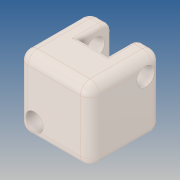
# Autodesk Inventor part: 方块2_beta
Saved by Autodesk Inventor 2019.1 (Build 231200000, 200)
## iProperties
Created: 2020-09-27
Part Number: 方块2_beta
Material: Generic
Document SubType Name: Modeling
Designer: 谢庆红冰
Density: 1 g/cm^3
Appearance: 缎光 - 亚麻
Author: 谢庆红冰
Autodesk Inventor part; units mm, degrees
ref_plane "YZ Plane" through (0, 0, 0) normal (1, 0, 0) x (0, 1, 0)
sketch "草图1" plane through (0, 0, 0) normal (0, 1, 0) x (-1, 0, 0)
  line L0 (-10, 10) -> (10, 10)
  line L1 (10, 10) -> (10, -10)
  line L2 (10, -10) -> (-10, -10)
  line L3 (-10, -10) -> (-10, 10)
  line L4 (-10, 10) -> (10, -10) construction
  line L5 (10, 10) -> (-10, -10) construction
  point P0 (0, 0)
  dimension "d0" = 20
  dimension "d1" = 20
  constraints: 12 end point, 2 midpoint, 2 parallel, 1 horizontal, 1 perpendicular
  measures "d0" distance of L0.end L1.end
  measures "d1" distance of L1.end L2.end
extrude "拉伸1" add sketch "草图1" along normal blind 20
ref_plane "工作平面1" through (0, 0, 10) normal (1, 0, 0) x (0, 0, -1)
sketch "草图6" plane through (0, 0, 0) normal (0, 0, 1) x (1, 0, 0)
  line L0 (10, 0) -> (-10, 0) construction
  line L1 (10, 0) -> (10, 20) construction
  line L2 (-10, 20) -> (10, 20) construction
  line L3 (-10, 0) -> (-10, 20) construction
  line L4 (-10, 20) -> (10, 0) construction
  line L5 (7.5, 12.5) -> (-2.5, 12.5)
  line L6 (-2.5, 12.5) -> (-2.5, 2.5)
  line L7 (-2.5, 2.5) -> (7.5, 2.5)
  line L8 (7.5, 2.5) -> (7.5, 12.5)
  line L9 (7.5, 12.5) -> (-2.5, 2.5) construction
  line L10 (-2.5, 12.5) -> (7.5, 2.5) construction
  point P0 (0, 0)
  point P1 (2.5, 7.5)
  dimension "d58" = 10
  dimension "d59" = 10
  constraints: 14 end point, 2 midpoint, 2 parallel, 1 horizontal, 1 perpendicular, 1 point on line
  measures "d58" distance of L7.end L6.end
  measures "d59" distance of L5.end L6.end
extrude "拉伸6" [suppressed]
sketch "草图2" plane through (0, 0, 10) normal (1, 0, 0) x (0, 0, -1)
  line L0 (20, 0) -> (0, 0) construction
  line L1 (20, 0) -> (20, 20) construction
  line L2 (0, 20) -> (20, 20) construction
  line L3 (0, 0) -> (0, 20) construction
  line L4 (20, 20) -> (20, 11)
  line L5 (20, 20) -> (11, 20)
  line L6 (20, 11) -> (11, 11)
  line L7 (11, 11) -> (11, 20)
  point P0 (10, 0)
  dimension "d4" = 9
  dimension "d5" = 9
  constraints: 9 end point, 2 perpendicular, 2 point on line
  measures "d4" distance of L4.end L1.end
  measures "d5" distance of L1.end L5.end
extrude "拉伸2" cut sketch "草图2" along normal mid plane 8
ref_plane "工作平面2" through (-10, 0, 0) normal (0, 0, 1) x (1, 0, 0)
sketch "草图3" plane through (-10, 0, 0) normal (0, 0, 1) x (1, 0, 0)
  line L0 (20, 0) -> (0, 0) construction
  line L1 (20, 0) -> (20, 20) construction
  line L2 (0, 20) -> (20, 20) construction
  line L3 (0, 0) -> (0, 20) construction
  line L4 (0, 0) -> (6, 0)
  line L5 (0, 0) -> (9, 0)
  line L6 (9, 0) -> (9, 9)
  line L7 (9, 9) -> (0, 9)
  line L8 (0, 9) -> (0, 0)
  point P0 (10, 0)
  dimension "d8" = 6
  dimension "d9" = 9
  dimension "d10" = 9
  constraints: 10 end point, 2 parallel, 1 horizontal, 1 perpendicular, 1 point on line
  measures "d8" distance of L0.end L4.end
  measures "d9" distance of L7.end L6.end
  measures "d10" distance of L5.end L6.end
extrude "拉伸3" cut sketch "草图3" along normal mid plane 8
sketch "草图4" plane through (-10, 0, 0) normal (0, 0, 1) x (1, 0, 0)
  line L0 (20, 0) -> (0, 0) construction
  line L1 (20, 0) -> (20, 20) construction
  line L2 (0, 20) -> (20, 20) construction
  line L3 (0, 0) -> (0, 20) construction
  line L4 (4.5, 6.5) -> (4.5, 2.5) construction
  line L5 (3.75, 5.75) -> (3.75, 3.25)
  arc A0 (3.75, 3.25) -> (5.25, 3.25) centre (4.5, 3.25) ccw
  arc A1 (5.25, 5.75) -> (3.75, 5.75) centre (4.5, 5.75) ccw
  line L6 (3.75, 5.75) -> (3.75, 3.25)
  line L7 (0, 0) -> (9, 0) construction
  line L8 (0, 9) -> (0, 0) construction
  line L9 (9, 9) -> (0, 9) construction
  line L10 (9, 0) -> (9, 9) construction
  line L11 (0, 9) -> (9, 0) construction
  line L12 (0, 0) -> (9.9155, 8.0845) construction
  line L13 (5.25, 3.25) -> (5.25, 5.75)
  line L14 (3.75, 5.75) -> (5.25, 5.75) construction
  line L15 (2.5, 4.5) -> (6.5, 4.5) construction
  line L16 (3.25, 3.75) -> (5.75, 3.75)
  line L17 (3.25, 3.75) -> (5.75, 3.75)
  arc A2 (5.75, 3.75) -> (5.75, 5.25) centre (5.75, 4.5) ccw
  arc A3 (3.25, 5.25) -> (3.25, 3.75) centre (3.25, 4.5) ccw
  line L18 (5.75, 5.25) -> (3.25, 5.25)
  line L19 (3.25, 3.75) -> (3.25, 5.25) construction
  circle A4 centre (4.5, 4.5) radius 2.5
  point P0 (10, 0)
  point P1 (3, 3)
  point P2 (3, 3)
  point P3 (3, 3)
  point P4 (4.5, 4.5)
  point P5 (3, 3)
  point P6 (3, 3)
  point P7 (3, 3)
  point P8 (3, 3)
  dimension "d42" = 0.75
  dimension "d43" = 0.75
  dimension "d44" = 2.5
  dimension "d45" = 1.5
  dimension "d46" = 0.75
  dimension "d47" = 0.75
  dimension "d48" = 2.5
  dimension "d49" = 1.5
  dimension "d66" = 5
  constraints: 24 end point, 12 point on circle, 5 centre point, 5 parallel, 4 point on line, 3 midpoint, 1 coincident, 1 horizontal
  measures "d42" radius of A1
  measures "d43" radius of A0
  measures "d44" distance of L13.start L13.end
  measures "d45" distance of L5.start L13.end
  measures "d46" radius of A3
  measures "d47" radius of A2
  measures "d48" distance of L18.start L19.end
  measures "d49" distance of L16.start L19.end
  measures "d66" diameter of A4
extrude "拉伸4" cut sketch "草图4" along normal through all both and the other way through all contours A1 L13 L18 L5 | L18 L13 L16 L5 | L5 L16 A3 L18 | L16 L13 A0 L5 | L18 A2 L16 L13 | A4
sketch "草图5" plane through (0, 0, 10) normal (1, 0, 0) x (0, 0, -1)
  line L0 (20, 0) -> (0, 0) construction
  line L1 (20, 0) -> (20, 20) construction
  line L2 (0, 20) -> (20, 20) construction
  line L3 (0, 0) -> (0, 20) construction
  line L4 (20, 20) -> (20, 11) construction
  line L5 (11, 20) -> (20, 20) construction
  line L6 (11, 11) -> (11, 20) construction
  line L7 (20, 11) -> (11, 11) construction
  line L8 (11, 20) -> (20, 11) construction
  line L9 (15.5, 17.5) -> (15.5, 13.5) construction
  line L10 (14.75, 16.75) -> (14.75, 14.25)
  line L11 (14.75, 16.75) -> (14.75, 14.25)
  arc A0 (14.75, 14.25) -> (16.25, 14.25) centre (15.5, 14.25) ccw
  arc A1 (16.25, 16.75) -> (14.75, 16.75) centre (15.5, 16.75) ccw
  line L12 (16.25, 14.25) -> (16.25, 16.75)
  line L13 (14.75, 16.75) -> (16.25, 16.75) construction
  line L14 (14.25, 14.75) -> (16.75, 14.75)
  line L15 (14.25, 14.75) -> (16.75, 14.75)
  line L16 (13.5, 15.5) -> (17.5, 15.5) construction
  line L17 (14.25, 14.75) -> (14.25, 16.25) construction
  line L18 (16.75, 16.25) -> (14.25, 16.25)
  arc A2 (16.75, 14.75) -> (16.75, 16.25) centre (16.75, 15.5) ccw
  arc A3 (14.25, 16.25) -> (14.25, 14.75) centre (14.25, 15.5) ccw
  line L19 (12.5, 12.5) -> (20, 20) construction
  circle A4 centre (15.5, 15.5) radius 2.5
  point P0 (10, 0)
  point P1 (7.5, 0)
  point P2 (3, 3)
  point P3 (3, 3)
  point P4 (3, 3)
  point P5 (3, 3)
  point P6 (3, 3)
  point P7 (3, 3)
  point P8 (3, 3)
  point P9 (3, 3)
  point P10 (16.25, 16.25)
  dimension "d50" = 0.75
  dimension "d51" = 0.75
  dimension "d52" = 2.5
  dimension "d53" = 1.5
  dimension "d54" = 0.75
  dimension "d55" = 0.75
  dimension "d56" = 2.5
  dimension "d57" = 1.5
  dimension "d65" = 5
  constraints: 24 end point, 12 point on circle, 5 centre point, 5 parallel, 4 midpoint, 4 point on line, 1 coincident, 1 horizontal
  measures "d50" radius of A1
  measures "d51" radius of A0
  measures "d52" distance of L12.start L12.end
  measures "d53" distance of L10.start L12.end
  measures "d54" radius of A3
  measures "d55" radius of A2
  measures "d56" distance of L18.start L18.end
  measures "d57" distance of L15.start L18.end
  measures "d65" diameter of A4
extrude "拉伸5" cut sketch "草图5" along normal through all both and the other way through all contours A1 L12 L18 L10 | L18 L12 L14 L10 | L10 L14 A3 L18 | L14 L12 A0 L10 | L18 A2 L14 L12 | A4
fillet "圆角1" radius 2.7 14 edges at (0, 20, 10) (10, 10, 10) (10, 0, 0) (10, 20, 0) (10, 10, -10) (0, 0, -10) (0, 0, 10) (-10, 0, 7) (-10, 0, -7) (-10, 10, -10) (-7, 20, -10) (7, 20, -10) (-10, 20, 0) (-10, 10, 10)
fillet "圆角2" [suppressed]
fillet "圆角3" radius 1 16 edges at (-1, 0, 0) (-9.2092, 0.7908, 4) (-10, 5.85, 4) (-4.15, 0, 4) (-10, 9, 0) (-10, 5.85, -4) (-4.15, 0, -4) (-9.2092, 0.7908, -4) (0, 11, -10) (4, 19.2092, -9.2092) (4, 20, -4.15) (4, 14.15, -10) (0, 20, -1) (-4, 19.2092, -9.2092) (-4, 20, -4.15) (-4, 14.15, -10)
fillet "圆角4" [suppressed]
sketch "草图7" plane through (10, 2.7, 7.3) normal (1, 0, 0) x (0, 0, -1)
  point P0 (7.3, -2.7)
  point P1 (12.8, 12.8)
sketch "草图8" plane through (-10, 2.7, 7.3) normal (-1, 0, 0) x (0, 0, 1)
  point P0 (-7.3, -2.7)
  point P1 (-7.75, 9)
  point P2 (-10.75, 9.5)
  point P3 (-12.8, 12.8)
sketch "草图9" plane through (7.3, 2.7, -10) normal (0, 0, -1) x (-1, 0, 0)
  point P0 (7.75, 1)
  point P1 (10.75, 1.5)
  point P2 (12.8, 1.8)
sketch "草图10" plane through (-7.3, 17.3, 10) normal (0, 0, 1) x (1, 0, 0)
  point P0 (2.25, -9)
  point P1 (0.25, -9.5)
  point P2 (1.8, -12.8)
